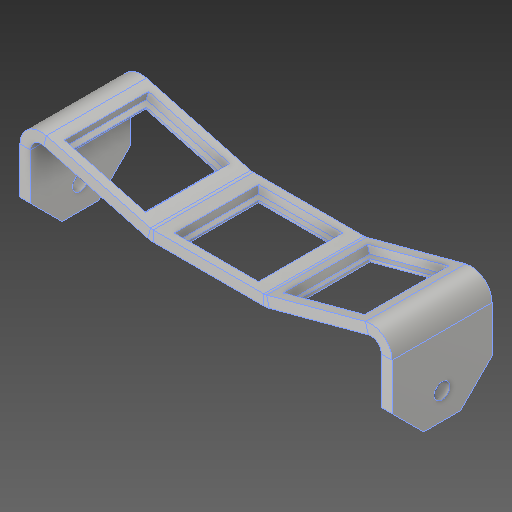
# Autodesk Inventor part: keyplate3
Saved by Autodesk Inventor 2018 (Build 220112000, 112)
## iProperties
Created: 2018-05-25
Part Number: keyplate3
Material: アルミニウム 6061
Document SubType Name: Sheet Metal
Designer: NaMACHAN
Density: 2.7 g/cm^3
Sheet Metal Rule: Al2mm
Appearance: アルミニウム - フラット
Mass: 6.17502 g
Surface Area: 34.4058 cm^2
Volume: 2.28704 cm^3
Flat Pattern Width: 1.9 cm
Flat Pattern Length: 10.2585 cm
Flat Pattern Area: 19.4911 cm^2
Sheet Metal Width: 19.000 mm
Sheet Metal Length: 102.585 mm
Sheet Metal Area: 1949.109 mm^2
Author: NaMACHAN
Autodesk Inventor part; units mm, degrees
ref_plane "YZ Plane" through (0, 0, 0) normal (1, 0, 0) x (0, 1, 0)
ref_plane "XZ Plane" through (0, 0, 0) normal (0, 1, 0) x (-1, 0, 0)
ref_plane "XY Plane" through (0, 0, 0) normal (0, 0, 1) x (1, 0, 0)
sketch "スケッチ1" plane through (0, 0, 0) normal (0, 1, 0) x (-1, 0, 0)
  line L0 (-10.5, -9.5) -> (10.5, -9.5)
  line L1 (10.5, -9.5) -> (10.5, 9.5)
  line L2 (10.5, 9.5) -> (-10.5, 9.5)
  line L3 (-10.5, 9.5) -> (-10.5, -9.5)
  line L4 (-10.5, -9.5) -> (10.5, 9.5) construction
  line L5 (10.5, -9.5) -> (-10.5, 9.5) construction
  line L6 (-7, -7) -> (7, -7)
  line L7 (7, -7) -> (7, 7)
  line L8 (7, 7) -> (-7, 7)
  line L9 (-7, 7) -> (-7, -7)
  line L10 (-7, -7) -> (7, 7) construction
  line L11 (7, -7) -> (-7, 7) construction
  point P0 (0, 0)
  dimension "d0" = 21
  dimension "d1" = 19
  dimension "d2" = 14
  dimension "d3" = 14
  measures "d0" distance of L2.end L1.end
  measures "d1" distance of L1.end L0.end
  measures "d2" distance of L8.end L7.end
  measures "d3" distance of L7.end L6.end
extrude "プレート1" add sketch "スケッチ1" along normal blind 2
sketch "スケッチ2" plane through (-11.0176, 2.0681, 9.5) normal (-0.258819, -0.9659258, 0) x (0.9659258, -0.258819, 0)
  line L0 (0, -19) -> (0, 0)
  line L1 (0, 0) -> (-20.4734, 0)
  line L2 (-20.4734, 0) -> (-20.4734, -19)
  line L3 (-20.4734, -19) -> (0, -19)
  constraints: 6 end point, 1 horizontal, 1 perpendicular, 1 vertical
edge flange "フランジ1" height 21 angle 15 thickness 2 bend radius 2 thickness toward (-0.258819, -0.9659258, 0) relief straight relief width 2 relief depth 1 edges at (-10.5, 2, 0) wall of the first edge with corners at (-11.0176, 2.0681, -9.5) (-11.0176, 2.0681, 9.5) (-30.7934, 7.3671, 9.5) (-30.7934, 7.3671, -9.5)
bend "曲げ1"
corner "コーナー1"
sketch "スケッチ9" plane through (-11.0176, 2.0681, 9.5) normal (0.258819, 0.9659258, 0) x (0.9659258, -0.258819, 0)
  line L0 (-17.5, 16.5) -> (-3.5, 16.5)
  line L1 (-3.5, 16.5) -> (-3.5, 2.5)
  line L2 (-3.5, 2.5) -> (-17.5, 2.5)
  line L3 (-17.5, 2.5) -> (-17.5, 16.5)
  line L4 (-17.5, 16.5) -> (-3.5, 2.5) construction
  line L5 (-3.5, 16.5) -> (-17.5, 2.5) construction
  line L6 (-20.4734, 0) -> (0, 0) projected
  line L7 (-20.4734, 19) -> (-20.4734, 0) projected
  line L8 (0, 0) -> (0, 19) projected
  point P0 (11.1775, 9.5)
  point P1 (-10.5, 9.5)
  point P2 (-10.5, 9.5)
  point P3 (-24.9734, 9.5)
  point P4 (-10.5, 9.5)
  point P5 (-10.2367, 0)
  point P6 (-17.5, 9.5)
  point P7 (-20.4734, 9.5)
  dimension "d63" = 14
  dimension "d64" = 14
  dimension "d204" = 10.5
  constraints: 12 end point, 6 midpoint, 2 horizontal alignment, 2 parallel, 1 horizontal, 1 perpendicular, 2 other
  measures "d63" distance of L1.end L2.end
  measures "d64" distance of L0.end L1.end
  measures "d204" distance from line of L8 point (-10.5, 9.5)
extrude "押し出し3" cut sketch "スケッチ9" against normal blind 10
sketch "スケッチ26" plane through (-33.8287, 3.5033, -9.5) normal (-1, 0, 0) x (0, -1, 0)
  line L0 (0, 19) -> (0, 0)
  line L1 (0, 0) -> (14.7871, 0)
  line L2 (14.7871, 0) -> (14.7871, 19)
  line L3 (14.7871, 19) -> (0, 19)
  constraints: 6 end point, 1 horizontal, 1 perpendicular, 1 vertical
edge flange "フランジ13" height 20 angle 105 thickness 2 bend radius 2 thickness toward (-1, 0, 0) relief straight relief width 2 relief depth 1 edges at (-31.3111, 5.4352, 0) wall of the first edge with corners at (-33.8287, 3.5033, 9.5) (-33.8287, 3.5033, -9.5) (-33.8287, -11.2838, -9.5) (-33.8287, -11.2838, 9.5)
bend "曲げ13"
corner "コーナー13"
sketch "スケッチ33" plane through (0, 2, 0) normal (0, 1, 0) x (1, 0, 0)
  line L0 (8, 8) -> (-8, 8)
  line L1 (-8, 8) -> (-8, -8)
  line L2 (-8, -8) -> (8, -8)
  line L3 (8, -8) -> (8, 8)
  line L4 (8, 8) -> (-8, -8) construction
  line L5 (-8, 8) -> (8, -8) construction
  point P0 (0, 0)
  dimension "d265" = 16
  dimension "d266" = 16
  constraints: 12 end point, 2 midpoint, 2 parallel, 1 horizontal, 1 perpendicular
  measures "d265" distance of L2.end L1.end
  measures "d266" distance of L1.end L0.end
extrude "押し出し11" cut sketch "スケッチ33" against normal blind 1.6
sketch "スケッチ34" plane through (-11.0176, 2.0681, 9.5) normal (0.258819, 0.9659258, 0) x (0.9659258, -0.258819, 0)
  line L0 (-2.5, 17.5) -> (-18.5, 17.5)
  line L1 (-18.5, 17.5) -> (-18.5, 1.5)
  line L2 (-18.5, 1.5) -> (-2.5, 1.5)
  line L3 (-2.5, 1.5) -> (-2.5, 17.5)
  line L4 (-2.5, 17.5) -> (-18.5, 1.5) construction
  line L5 (-18.5, 17.5) -> (-2.5, 1.5) construction
  line L6 (-17.5, 2.5) -> (-17.5, 16.5) projected
  line L7 (-17.5, 16.5) -> (-3.5, 16.5) projected
  point P0 (11.1775, 9.5)
  point P1 (-10.5, 9.5)
  point P2 (-10.5, 9.5)
  point P3 (-17.5, 9.5)
  point P4 (-10.5, 9.5)
  point P5 (-10.5, 16.5)
  dimension "d269" = 16
  dimension "d270" = 16
  constraints: 12 end point, 6 midpoint, 2 parallel, 1 horizontal, 1 horizontal alignment, 1 perpendicular, 1 vertical alignment
  measures "d269" distance of L2.end L1.end
  measures "d270" distance of L1.end L0.end
extrude "押し出し12" cut sketch "スケッチ34" against normal blind 1.6
sketch "スケッチ36" plane through (11.0176, 2.0681, -9.5) normal (0.258819, -0.9659258, 0) x (0.9659258, 0.258819, 0)
  line L0 (0, 19) -> (0, 0)
  line L1 (0, 0) -> (19.4734, 0)
  line L2 (19.4734, 0) -> (19.4734, 19)
  line L3 (19.4734, 19) -> (0, 19)
  constraints: 6 end point, 1 horizontal, 1 perpendicular, 1 vertical
edge flange "フランジ16" height 20 angle 15 thickness 2 bend radius 2 thickness toward (0.258819, -0.9659258, 0) relief straight relief width 2 relief depth 1 edges at (10.5, 2, 0) wall of the first edge with corners at (11.0176, 2.0681, 9.5) (11.0176, 2.0681, -9.5) (29.8275, 7.1082, -9.5) (29.8275, 7.1082, 9.5)
bend "曲げ17"
corner "コーナー16"
sketch "スケッチ37" plane through (32.8628, 3.2445, 9.5) normal (1, 0, 0) x (0, 1, 0)
  line L0 (0, -19) -> (0, 0)
  line L1 (0, 0) -> (-14.7871, 0)
  line L2 (-14.7871, 0) -> (-14.7871, -19)
  line L3 (-14.7871, -19) -> (0, -19)
  constraints: 6 end point, 1 horizontal, 1 perpendicular, 1 vertical
edge flange "フランジ17" height 20 angle 105 thickness 2 bend radius 2 thickness toward (1, 0, 0) relief straight relief width 2 relief depth 1 edges at (30.3451, 5.1764, 0) wall of the first edge with corners at (32.8628, 3.2445, -9.5) (32.8628, 3.2445, 9.5) (32.8628, -11.5426, 9.5) (32.8628, -11.5426, -9.5)
bend "曲げ18"
corner "コーナー17"
sketch "スケッチ38" plane through (11.0176, 2.0681, 9.5) normal (-0.258819, 0.9659258, 0) x (0.9659258, 0.258819, 0)
  line L0 (16.7367, 2.5) -> (2.7367, 2.5)
  line L1 (2.7367, 2.5) -> (2.7367, 16.5)
  line L2 (2.7367, 16.5) -> (16.7367, 16.5)
  line L3 (16.7367, 16.5) -> (16.7367, 2.5)
  line L4 (16.7367, 2.5) -> (2.7367, 16.5) construction
  line L5 (2.7367, 2.5) -> (16.7367, 16.5) construction
  line L6 (19.4734, 0) -> (19.4734, 19) projected
  line L7 (19.4734, 19) -> (0, 19) projected
  point P0 (-11.1775, 9.5)
  point P1 (9.7367, 9.5)
  point P2 (9.7367, 9.5)
  point P3 (19.4734, 9.5)
  point P4 (9.7367, 9.5)
  point P5 (9.7367, 19)
  dimension "d298" = 14
  dimension "d299" = 14
  constraints: 12 end point, 6 midpoint, 2 parallel, 1 horizontal, 1 horizontal alignment, 1 perpendicular, 1 vertical alignment
  measures "d298" distance of L1.end L2.end
  measures "d299" distance of L0.end L1.end
extrude "押し出し14" cut sketch "スケッチ38" against normal blind 10
sketch "スケッチ39" plane through (11.0176, 2.0681, 9.5) normal (-0.258819, 0.9659258, 0) x (0.9659258, 0.258819, 0)
  line L0 (17.7367, 1.5) -> (1.7367, 1.5)
  line L1 (1.7367, 1.5) -> (1.7367, 17.5)
  line L2 (1.7367, 17.5) -> (17.7367, 17.5)
  line L3 (17.7367, 17.5) -> (17.7367, 1.5)
  line L4 (17.7367, 1.5) -> (1.7367, 17.5) construction
  line L5 (1.7367, 1.5) -> (17.7367, 17.5) construction
  line L6 (23.3371, 19) -> (23.3371, 0) projected
  line L7 (19.4734, 19) -> (0, 19) projected
  point P0 (-11.1775, 9.5)
  point P1 (9.7367, 9.5)
  point P2 (9.7367, 9.5)
  point P3 (23.3371, 9.5)
  point P4 (9.7367, 9.5)
  point P5 (9.7367, 19)
  dimension "d302" = 16
  dimension "d303" = 16
  constraints: 12 end point, 6 midpoint, 2 parallel, 1 horizontal, 1 horizontal alignment, 1 perpendicular, 1 vertical alignment
  measures "d302" distance of L1.end L2.end
  measures "d303" distance of L0.end L1.end
extrude "押し出し15" cut sketch "スケッチ39" against normal blind 1.5
sketch "スケッチ40" plane through (-35.8287, 3.5033, -9.5) normal (-1, 0, 0) x (0, 0, 1)
  line L0 (19, -14.7871) -> (0, -14.7871) projected
  line L1 (0, -15.0459) -> (19, -15.0459) projected
  point P0 (9.5, -3.5033)
  point P1 (9.5, -10.0459)
  point P2 (9.5, -14.7871)
  point P3 (13, -14.7871)
  point P4 (6, -14.7871)
  dimension "d306" = 5
  constraints: 1 midpoint, 1 vertical alignment
  measures "d306" distance from line of L1 point (9.5, -10.046)
hole "穴6" at (-35.8287, -6.5426, 0) direction (1, 0, 0) diameter 3 end through all
chamfer "コーナー面取り1" distance 6 angle 45 4 edges at (-34.8287, -11.2838, 9.5) (-34.8287, -11.2838, -9.5) (33.8628, -11.5426, 9.5) (33.8628, -11.5426, -9.5)
equation "\"d4\" = Thickness"
equation "\"d5\" = BendReliefWidth"
equation "\"d6\" = BendReliefDepth"
equation "\"d7\" = MinimumRemnant"
equation "\"d8\" = TransitionRadius"
equation "\"d11\" = BendRadius"
equation "\"d12\" = CornerReliefSize"
equation "\"d13\" = GapSize"
equation "\"d14\" = JacobiRadiusSize"
equation "\"d205\" = BendReliefWidth"
equation "\"d206\" = BendReliefDepth"
equation "\"d207\" = MinimumRemnant"
equation "\"d208\" = TransitionRadius"
equation "\"d211\" = BendRadius"
equation "\"d212\" = CornerReliefSize"
equation "\"d213\" = GapSize"
equation "\"d214\" = JacobiRadiusSize"
equation "\"d278\" = BendReliefWidth"
equation "\"d279\" = BendReliefDepth"
equation "\"d280\" = MinimumRemnant"
equation "\"d281\" = TransitionRadius"
equation "\"d284\" = BendRadius"
equation "\"d285\" = CornerReliefSize"
equation "\"d286\" = GapSize"
equation "\"d287\" = JacobiRadiusSize"
equation "\"d288\" = BendReliefWidth"
equation "\"d289\" = BendReliefDepth"
equation "\"d290\" = MinimumRemnant"
equation "\"d291\" = TransitionRadius"
equation "\"d294\" = BendRadius"
equation "\"d295\" = CornerReliefSize"
equation "\"d296\" = GapSize"
equation "\"d297\" = JacobiRadiusSize"
equation "\"BendRadius\" = Thickness"
equation "\"BendReliefWidth\" = Thickness"
equation "\"BendReliefDepth\" = 0.5 * Thickness"
equation "\"CornerReliefSize\" = 4 * Thickness"
equation "\"MinimumRemnant\" = 2 * Thickness"
equation "\"TransitionRadius\" = BendRadius"
equation "\"JacobiRadiusSize\" = BendRadius"
equation "\"GapSize\" = Thickness"
equation "\"Thickness\" = 2"
